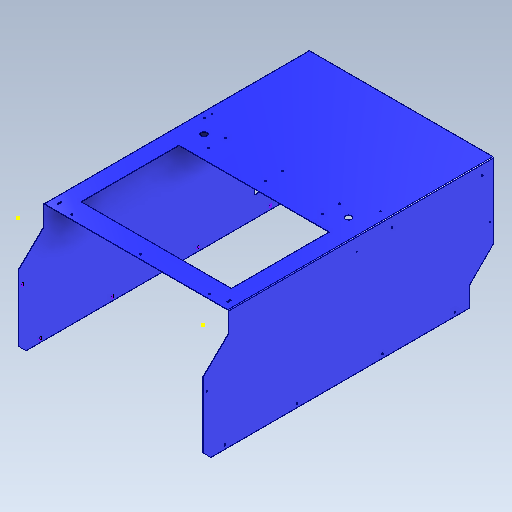
# Autodesk Inventor part: Carcasa_azul
Saved by Autodesk Inventor 2021 (Build 250183000, 183)
## iProperties
Created: 2021-04-15
Part Number: Carcasa_azul
Material: Acero AISI 1006 85 LC
Document SubType Name: Chapa
Designer: Admin
Density: 7.872 g/cm^3
Sheet Metal Rule: Por defecto_mm
Appearance: Acero
Mass: 7759.46 g
Surface Area: 16366.1 cm^2
Volume: 985.703 cm^3
Flat Pattern Width: 83.1 cm
Flat Pattern Length: 120.579 cm
Flat Pattern Area: 10020.1 cm^2
Sheet Metal Width: 831,000 mm
Sheet Metal Length: 1205,794 mm
Sheet Metal Area: 1002014,740 mm^2
Author: Admin
Autodesk Inventor part; units mm, degrees
ref_plane "YZ Plane" through (0, 0, 0) normal (1, 0, 0) x (0, 1, 0)
ref_plane "XZ Plane" through (0, 0, 0) normal (0, 1, 0) x (-1, 0, 0)
ref_plane "XY Plane" through (0, 0, 0) normal (0, 0, 1) x (1, 0, 0)
sketch "Boceto1" plane through (0, 0, 0) normal (0, 1, 0) x (-1, 0, 0)
  line L0 (0, 0) -> (530, 0)
  line L1 (530, 0) -> (530, -831)
  line L2 (530, -831) -> (0, -831)
  line L3 (0, -831) -> (0, 0)
  dimension "d0" = 530
  dimension "d1" = 831
  measures "d0" distance of L1.end L2.end
  measures "d1" distance of L0.end L1.end
extrude "Placa1" add sketch "Boceto1" along normal blind 1.21
sketch "Boceto2" plane through (-1.21, 1.21, -831) normal (1, 0, 0) x (0, -1, 0)
  line L0 (0, 831) -> (0, 0)
  line L1 (0, 0) -> (340, 0)
  line L2 (340, 0) -> (340, 831)
  line L3 (340, 831) -> (0, 831)
  constraints: 6 end point, 1 horizontal, 1 perpendicular, 1 vertical
edge flange "Pestaña1" height 340 angle 90 thickness 1.21 bend radius 1.21 thickness toward (1, 0, 0) relief straight relief width 1.21 relief depth 0.605 edges at (0, 1.21, -415.5) wall of the first edge with corners at (-1.21, 1.21, 0) (-1.21, 1.21, -831) (-1.21, -338.79, -831) (-1.21, -338.79, 0)
bend "Doblez1"
corner "Esquina1"
sketch "Boceto3" plane through (-528.79, 1.21, 0) normal (-1, 0, 0) x (0, 1, 0)
  line L0 (0, -831) -> (0, 0)
  line L1 (0, 0) -> (-340, 0)
  line L2 (-340, 0) -> (-340, -831)
  line L3 (-340, -831) -> (0, -831)
  constraints: 6 end point, 1 horizontal, 1 perpendicular, 1 vertical
edge flange "Pestaña2" height 340 angle 90 thickness 1.21 bend radius 1.21 thickness toward (-1, 0, 0) relief straight relief width 1.21 relief depth 0.605 edges at (-530, 1.21, -415.5) wall of the first edge with corners at (-528.79, 1.21, -831) (-528.79, 1.21, 0) (-528.79, -338.79, 0) (-528.79, -338.79, -831)
bend "Doblez2"
corner "Esquina2"
sketch "Boceto4" plane through (-530, -338.79, -831) normal (-1, 0, 0) x (0, 0, 1)
  line L0 (0, 337.58) -> (0, 0) projected
  line L1 (831, 0) -> (0, 0) projected
  line L2 (70, 0) -> (70, 56.2)
  line L3 (0, 340) -> (0, 338.79) projected
  line L4 (0, 340) -> (0, 126)
  line L5 (70, 56.2) -> (0, 126)
  line L6 (831, 337.58) -> (831, 0) projected
  line L7 (831, 0) -> (809.4, 0)
  line L8 (831, 0) -> (758.8, 0)
  line L9 (831, 340) -> (0, 340) projected
  line L10 (758.8, 340) -> (758.8, 281)
  line L11 (758.8, 281) -> (831, 211)
  line L12 (809.4, 0) -> (831, 21.6)
  line L13 (758.8, 340) -> (831, 340)
  line L14 (831, 211) -> (831, 340)
  point P0 (831, 338.79)
  dimension "d23" = 70
  dimension "d24" = 56.2
  dimension "d25" = 214
  dimension "d26" = 21.6
  dimension "d28" = 72.2
  dimension "d29" = 59
  constraints: 20 end point, 7 point on line, 1 collinear, 1 horizontal, 1 vertical
  measures "d23" distance of L0.end L2.start
  measures "d24" distance of L2.start L2.end
  measures "d25" distance of L3.start L4.end
  measures "d26" distance of L1.start L7.end
  measures "d28" distance of L1.start L8.end
  measures "d29" distance of L10.start L10.end
extrude "Extrusión1" cut sketch "Boceto4" against normal through all contours L5 L2 L1 L0 | L9 L14 L6 L11 L10 | L12 L6 L1
sketch "Boceto5" plane through (0, 1.21, 0) normal (0, 1, 0) x (1, 0, 0)
  line L0 (-527.58, 72.2) -> (-2.42, 72.2) projected
  line L1 (-265, 0) -> (-265, 130)
  line L2 (-265, 130) -> (-50, 130)
  line L3 (-265, 130) -> (-480, 130)
  line L4 (-480, 130) -> (-480, 410)
  line L5 (-480, 410) -> (-50, 410)
  line L6 (-50, 410) -> (-50, 130)
  point P0 (0, 0)
  dimension "d33" = 130
  dimension "d34" = 215
  dimension "d35" = 215
  dimension "d36" = 280
  dimension "d37" = 430
  constraints: 12 end point, 2 horizontal, 2 perpendicular
  measures "d33" distance of L1.start L1.end
  measures "d34" distance of L1.end L2.end
  measures "d35" distance of L1.end L3.end
  measures "d36" distance of L3.end L4.end
  measures "d37" distance of L4.end L5.end
extrude "Extrusión2" cut sketch "Boceto5" against normal through all
sketch "Boceto6" plane through (-530, -212.79, -831) normal (-1, 0, 0) x (0, 0, 1)
  line L0 (70, -126) -> (70, -69.8) projected
  line L1 (70, -126) -> (132, -126)
  line L2 (70, -126) -> (809.4, -126) projected
  line L3 (132, -126) -> (132, -51)
  line L4 (109.15, -35.15) -> (154.85, -35.15)
  line L5 (154.85, -35.15) -> (154.85, -66.85)
  line L6 (154.85, -66.85) -> (109.15, -66.85)
  line L7 (109.15, -66.85) -> (109.15, -35.15)
  line L8 (109.15, -35.15) -> (154.85, -66.85) construction
  line L9 (154.85, -35.15) -> (109.15, -66.85) construction
  point P0 (831, 212.79)
  dimension "d40" = 62
  dimension "d41" = 75
  dimension "d42" = 45.7
  dimension "d43" = 31.7
  constraints: 16 end point, 2 midpoint, 2 parallel, 2 perpendicular, 1 horizontal, 1 point on line
  measures "d40" distance of L0.start L1.end
  measures "d41" distance of L1.end L3.end
  measures "d42" distance of L5.end L6.end
  measures "d43" distance of L4.end L5.end
extrude "Extrusión3" cut sketch "Boceto6" against normal blind 10
sketch "Boceto7" plane through (-530, -212.79, -831) normal (-1, 0, 0) x (0, 0, 1)
  arc A0 (130.7904, 7.8142) -> (133.2041, 7.8151) centre (132, 0) ccw
  line L0 (133.2041, 7.7745) -> (133.2041, 8.6263)
  line L1 (133.2041, 8.6263) -> (130.7904, 8.6263)
  line L2 (130.7904, 8.6263) -> (130.7904, 7.8142)
  line L3 (109.15, -66.85) -> (109.15, -35.15) projected
  line L4 (109.15, -35.15) -> (154.85, -35.15) projected
  line L5 (109.15, -66.85) -> (154.85, -35.15)
  line L6 (154.85, -35.15) -> (154.85, -66.85)
  line L7 (154.85, -66.85) -> (109.15, -35.15)
  point P0 (831, 212.79)
  point P1 (-1, -8.7)
  point P2 (1, -8.7)
  constraints: 10 end point, 2 point on circle, 1 centre point, 1 perpendicular, 1 point on line, 1 vertical, 3 other
extrude "Extrusión4" cut sketch "Boceto7" against normal blind 10 contours L2 L1 L0 A0
sketch "Boceto8" plane through (0, 1.21, 0) normal (0, 1, 0) x (1, 0, 0)
  line L0 (-50, 410) -> (-480, 410) projected
  line L1 (-73.0212, 410) -> (-9.5212, 410) construction
  line L2 (0, 21.6) -> (0, 761) projected
  line L3 (0, 473.5) -> (58.4, 473.5) construction
  circle A0 centre (-58.4, 473.5) radius 8.75
  line L4 (-527.58, 831) -> (-2.42, 831) projected
  circle A1 centre (-471.6, 473.5) radius 8.75
  line L5 (-480, 410) -> (-480, 130) projected
  point P0 (0, 0)
  dimension "d53" = 17.5
  constraints: 4 end point, 2 centre point, 2 horizontal, 2 point on line
  measures "d53" diameter of A0
extrude "Extrusión5" cut sketch "Boceto8" against normal through all
sketch "Boceto10" plane through (0, 1.21, 0) normal (0, 1, 0) x (1, 0, 0)
  circle A0 centre (-471.6, 473.5) radius 8.75 projected
  line L0 (-471.6, 473.5) -> (-471.6, 452.5)
  circle A1 centre (-58.4, 473.5) radius 8.75 projected
  line L1 (-58.4, 473.5) -> (-58.4, 452.5)
  line L2 (-471.6, 452.5) -> (-58.4, 452.5)
  line L3 (-50, 410) -> (-480, 410) projected
  line L4 (-490, 120) -> (-40, 120) construction
  line L5 (-480, 410) -> (-480, 130) projected
  line L6 (-40, 120) -> (410, 120) construction
  circle A2 centre (-471.6, 473.5) radius 17
  line L7 (-265, 452.5) -> (-508.79, 452.5)
  circle A3 centre (-58.4, 473.5) radius 17
  line L8 (-454.6, 473.5) -> (-75.4, 473.5)
  line L9 (-1.0392, 452.5) -> (-21.0392, 452.5)
  line L10 (-2.42, 72.2) -> (-2.42, 831) projected
  line L11 (-1.0392, 452.5) -> (18.9608, 452.5) construction
  line L12 (-35, 425) -> (-495, 425)
  line L13 (-495, 425) -> (-495, 115)
  line L14 (-495, 115) -> (-35, 115)
  line L15 (-35, 115) -> (-35, 425)
  line L16 (-35, 425) -> (-495, 115) construction
  line L17 (-495, 425) -> (-35, 115) construction
  line L18 (-35, 425) -> (425, 425) construction
  point P0 (0, 0)
  point P1 (-265, 270)
  dimension "d64" = 34
  dimension "d67" = 34
  dimension "d56" = 21
  dimension "d57" = 21
  dimension "d65" = 243.79
  dimension "d68" = 20
  dimension "d69" = 180
  dimension "d70" = 460
  dimension "d71" = 180
  dimension "d72" = 310
  constraints: 32 end point, 6 horizontal, 3 midpoint, 2 coincident, 2 collinear, 2 horizontal alignment, 2 parallel, 2 perpendicular, 2 vertical, 1 point on line, 4 other
  measures "d56" distance of L0.start L0.end
  measures "d57" distance of L1.start L1.end
  measures "d65" distance of L7.start L7.end
  measures "d68" distance of L9.start L9.end
  measures "d69" angle of L9 L11
  measures "d70" distance of L12.start L12.end
  measures "d71" angle of L12 L18
  measures "d72" distance of L13.end L12.end
sketch "Boceto11" plane through (-1.21, -212.79, -831) normal (-1, 0, 0) x (0, 0, 1)
  line L0 (70, -69.8) -> (70, -126) projected
  line L1 (70, -126) -> (390, -126)
  line L2 (809.4, -126) -> (70, -126) projected
  line L3 (390, -126) -> (390, -82.4489)
  point P0 (831, 212.79)
  dimension "d73" = 320
  constraints: 4 end point, 1 point on line, 1 vertical
  measures "d73" distance of L0.end L1.end
ref_plane "Plano de trabajo1" through (-1.21, -338.79, -441) normal (0, 0, 1) x (0, 1, 0)
sketch "Boceto12" plane through (0, 1.21, 0) normal (0, 1, 0) x (1, 0, 0)
  line L0 (-35.8569, 95.75) -> (-9.1431, 95.75) construction
  line L1 (-520.8569, 95.75) -> (-494.1431, 95.75) construction
  line L2 (-507.5, 91.75) -> (-507.5, 99.75) construction
  line L3 (-505.9125, 91.75) -> (-505.9125, 99.75)
  line L4 (-509.0875, 99.75) -> (-509.0875, 91.75)
  arc A0 (-509.0875, 91.75) -> (-505.9125, 91.75) centre (-507.5, 91.75) ccw
  arc A1 (-505.9125, 99.75) -> (-509.0875, 99.75) centre (-507.5, 99.75) ccw
  line L5 (-22.5, 91.75) -> (-22.5, 99.75) construction
  line L6 (-20.9125, 91.75) -> (-20.9125, 99.75)
  line L7 (-24.0875, 99.75) -> (-24.0875, 91.75)
  arc A2 (-24.0875, 91.75) -> (-20.9125, 91.75) centre (-22.5, 91.75) ccw
  arc A3 (-20.9125, 99.75) -> (-24.0875, 99.75) centre (-22.5, 99.75) ccw
  point P0 (0, 0)
  dimension "d78" = 3.175
  dimension "d80" = 3.175
  constraints: 20 end point, 8 point on circle, 8 tangent, 4 centre point, 2 horizontal, 2 parallel, 2 perpendicular
  measures "d78" diameter of A1
  measures "d80" diameter of A3
extrude "Cortar1" cut sketch "Boceto12" against normal blind 1.21
sketch "Boceto15" plane through (0, 1.21, 0) normal (0, 1, 0) x (1, 0, 0)
  line L0 (-527.58, 831) -> (-527.58, 72.2) projected
  line L1 (-527.58, 84.9) -> (-2.42, 84.9)
  line L2 (-2.42, 831) -> (-2.42, 72.2) projected
  line L3 (-527.58, 84.9) -> (-2.42, 84.9) construction
  line L4 (-527.58, 72.2) -> (-2.42, 72.2) projected
  line L5 (-527.58, 84.9) -> (-461.935, 84.9) construction
  line L6 (-527.58, 84.9) -> (-265, 84.9) construction
  line L7 (-2.42, 84.9) -> (-68.065, 84.9) construction
  circle A0 centre (-461.935, 84.9) radius 2.5
  circle A1 centre (-265, 84.9) radius 2.5
  circle A2 centre (-68.065, 84.9) radius 2.5
  point P0 (0, 0)
  dimension "d88" = 12.7
  dimension "d89" = 65.645
  dimension "d90" = 262.58
  dimension "d91" = 65.645
  dimension "d92" = 5
  dimension "d93" = 5
  dimension "d94" = 5
  constraints: 10 end point, 4 point on line, 3 centre point, 3 coincident, 1 collinear, 1 horizontal, 1 midpoint
  measures "d88" distance between parallel lines of L4 L1
  measures "d89" distance of L1.start L5.end
  measures "d90" distance of L1.start L6.end
  measures "d91" distance of L3.end L7.end
  measures "d92" diameter of A0
  measures "d93" diameter of A1
  measures "d94" diameter of A2
extrude "Cortar4" cut sketch "Boceto15" against normal blind 1.21 contours A0 L1 | L1 A0 | A1 L1 | L1 A1 | A2 L1 | L1 A2
sketch "Boceto17" plane through (0, 1.21, 0) normal (0, 1, 0) x (1, 0, 0)
  circle A0 centre (-511.08, 534.92) radius 1.5875 projected
  circle A1 centre (-27.7, 534.92) radius 1.5875 projected
  point P0 (0, 0)
extrude "Cortar6" cut sketch "Boceto17" against normal blind 1.21
sketch "Boceto18" plane through (0, -212.79, -831) normal (1, 0, 0) x (0, 0, -1)
  circle A0 centre (-392.4294, 174.69) radius 1.5875 projected
  point P0 (-831, 212.79)
extrude "Cortar7" cut sketch "Boceto18" against normal blind 1.21
sketch "Boceto19" plane through (-528.79, -212.79, -831) normal (1, 0, 0) x (0, 0, -1)
  circle A0 centre (-392.4294, 174.69) radius 1.5875 projected
  point P0 (-831, 212.79)
extrude "Cortar8" cut sketch "Boceto19" against normal blind 1.21
sketch "Boceto22" plane through (-530, -212.79, -831) normal (-1, 0, 0) x (0, 0, 1)
  circle A0 centre (110.83, -114.94) radius 2.5 projected
  circle A1 centre (317.98, -114.94) radius 2.5 projected
  circle A2 centre (562.63, -114.94) radius 2.5 projected
  circle A3 centre (769.18, -114.94) radius 2.5 projected
  circle A4 centre (820.66, 44.306) radius 2.5 projected
  circle A5 centre (110.83, -114.94) radius 2.5
  circle A6 centre (317.98, -114.94) radius 2.5
  circle A7 centre (562.63, -114.94) radius 2.5
  circle A8 centre (769.18, -114.94) radius 2.5
  circle A9 centre (820.66, 44.306) radius 2.5
  circle A10 centre (10.4246, 57.9426) radius 1.45
  point P0 (831, 212.79)
  dimension "d124" = 2.9
  constraints: 6 centre point, 4 coincident
  measures "d124" diameter of A10
extrude "Extrusión6" cut sketch "Boceto22" against normal through all contours A0 | A1 | A2 | A3 | A4
sketch "Boceto23" plane through (0, 1.21, 0) normal (0, 1, 0) x (1, 0, 0)
  point P0 (0, 0)
extrude "Extrusión7" cut sketch "Boceto22" against normal through all contours A10
sketch "Sketch24" plane through (0, 1.21, 0) normal (0, 1, 0) x (1, 0, 0)
  circle A0 centre (-511.29, 513.75) radius 1.5 projected
  circle A1 centre (-511.29, 513.75) radius 2
  point P0 (0, 0)
  dimension "d127" = 4
  constraints: 1 centre point, 1 coincident
  measures "d127" diameter of A1
extrude "Extrusion8" cut sketch "Sketch24" against normal up to next contours A0 | A1
sketch "Boceto26" plane through (0, 1.21, 0) normal (0, 1, 0) x (1, 0, 0)
  circle A0 centre (-104.99, 445.0706) radius 1.5875 projected
  line L0 (-104.99, 445.0706) -> (-48.19, 445.0706) construction
  circle A1 centre (-104.99, 495.0706) radius 2.5
  circle A2 centre (-268.29, 495.0706) radius 2.5
  circle A3 centre (-431.59, 495.0706) radius 2.5
  point P0 (0, 0)
  dimension "d133" = 50
  dimension "d134" = 163.3
  dimension "d135" = 163.3
  dimension "d136" = 5
  dimension "d137" = 5
  dimension "d138" = 5
  constraints: 3 centre point, 3 coincident, 2 end point, 1 horizontal
  measures "d133" distance of point (-104.99, 495.071) L0.start
  measures "d134" distance of point (-268.29, 495.071) point (-104.99, 495.071)
  measures "d135" distance of point (-431.59, 495.071) point (-268.29, 495.071)
  measures "d136" diameter of A1
  measures "d137" diameter of A2
  measures "d138" diameter of A3
extrude "Extrusión9" cut sketch "Boceto26" against normal through all contours A1 | A2 | A3
sketch "Boceto27" plane through (0, 1.21, 0) normal (0, 1, 0) x (1, 0, 0)
  circle A0 centre (-104.99, 445.0706) radius 2.5 projected
  circle A1 centre (-268.29, 445.0706) radius 2.5 projected
  circle A2 centre (-431.59, 445.0706) radius 2.5 projected
  point P0 (0, 0)
extrude "Extrusión10" cut sketch "Boceto27" against normal blind 5
thread "Rosca1" size "M5x0.8" class "6H" standard "ANSI Metric M Profile" length 16
thread "Rosca2" size "M5x0.8" class "6H" standard "ANSI Metric M Profile" length 16
thread "Rosca3" size "M5x0.8" class "6H" standard "ANSI Metric M Profile" length 16
sketch "Boceto28" plane through (-530, -212.79, -831) normal (-1, 0, 0) x (0, 0, 1)
  circle A0 centre (290.99, 184.5) radius 2.5 projected
  circle A1 centre (32.99, 184.5) radius 2.5 projected
  point P0 (831, 212.79)
extrude "Extrusión11" cut sketch "Boceto28" against normal through all
equation "\"d81\" = Grosor"
equation "\"d95\" = Grosor"
equation "\"d99\" = Grosor"
equation "\"d101\" = Grosor"
equation "\"d103\" = Grosor"
equation "\"d137\" = d136"
equation "\"d138\" = d136"
equation "\"d2\" = Grosor"
equation "\"d3\" = Anchura_desahogo_plegado"
equation "\"d4\" = Profundidad_desahogo_plegado"
equation "\"d5\" = Remanente_mínimo"
equation "\"d6\" = Radiodetransición"
equation "\"d9\" = Radio_pliegue"
equation "\"d10\" = Tamaño_destalonado"
equation "\"d11\" = TamañoSeparación"
equation "\"d12\" = Tamaño_de_radio_de_Jacobi"
equation "\"d13\" = Anchura_desahogo_plegado"
equation "\"d14\" = Profundidad_desahogo_plegado"
equation "\"d15\" = Remanente_mínimo"
equation "\"d16\" = Radiodetransición"
equation "\"d19\" = Radio_pliegue"
equation "\"d20\" = Tamaño_destalonado"
equation "\"d21\" = TamañoSeparación"
equation "\"d22\" = Tamaño_de_radio_de_Jacobi"
equation "\"Radio_pliegue\" = Grosor"
equation "\"Anchura_desahogo_plegado\" = Grosor"
equation "\"Profundidad_desahogo_plegado\" = 0.5 * Grosor"
equation "\"Tamaño_destalonado\" = 4 * Grosor"
equation "\"Remanente_mínimo\" = 2 * Grosor"
equation "\"Radiodetransición\" = Radio_pliegue"
equation "\"Tamaño_de_radio_de_Jacobi\" = Radio_pliegue"
equation "\"TamañoSeparación\" = Grosor"
equation "\"Grosor\" = 1.21"
